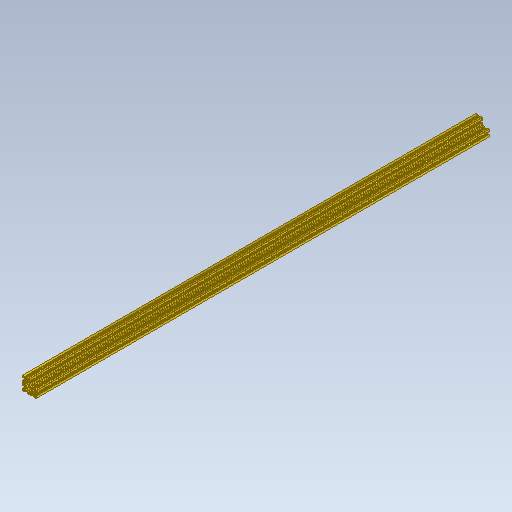
# Autodesk Inventor part: Perfil 60×60 L 8 rasgos_AST060060L08
Saved by Autodesk Inventor 2025.2 (Build 292293000, 293)
## iProperties
Created: 2025-04-07
Part Number: Perfil 60×60 L 8 rasgos_AST060060L08
Material: Ouro
Document SubType Name: Modeling
Designer: Gustavo Sousa
Density: 19.3 g/cm^3
Appearance: Metal quente 2400F
Author: Gustavo Sousa
Autodesk Inventor part; units mm, degrees
ref_plane "YZ Plane" through (0, 0, 0) normal (1, 0, 0) x (0, 1, 0)
ref_plane "XZ Plane" through (0, 0, 0) normal (0, 1, 0) x (-1, 0, 0)
ref_plane "XY Plane" through (0, 0, 0) normal (0, 0, 1) x (1, 0, 0)
sketch "Esboço1" plane through (0, 0, 0) normal (0, 0, 1) x (1, 0, 0)
  line L0 (-30, 30) -> (30, 30) construction
  line L1 (-30, 30) -> (-30, -30) construction
  line L2 (-30, -30) -> (30, -30) construction
  line L3 (30, 30) -> (30, -30) construction
  circle A0 centre (-15, 15) radius 5
  line L4 (-15, 15) -> (0, 0) construction
  line L5 (-15, 15) -> (0, 30) construction
  line L6 (-15, 15) -> (-30, 30) construction
  line L7 (-15, 15) -> (-30, 0) construction
  circle A1 centre (-26.5, 26.5) radius 2.25
  arc A2 (-29.5, 30) -> (-30, 29.5) centre (-29.5, 29.5) ccw
  line L8 (-22, 22) -> (-8, 22) construction
  line L9 (-19.1, 30) -> (-10.9, 30) construction
  line L10 (-19.1, 30) -> (-19.6, 30) construction
  line L11 (-19.6, 30) -> (-19.6, 29.5)
  line L12 (-19.6, 29.5) -> (-19.1, 29.5)
  line L13 (-19.1, 29.5) -> (-19.1, 30) construction
  line L14 (-19.6, 30) -> (-29.5, 30)
  line L15 (-19.1, 30) -> (-19.1, 27.8) construction
  line L16 (-19.1, 27.8) -> (-23.15, 27.8)
  line L17 (-19.1, 29.5) -> (-19.1, 27.8)
  line L18 (-22, 22) -> (-22, 8) construction
  line L19 (-23.15, 27.8) -> (-23.15, 24.7056)
  line L20 (-23.15, 24.7056) -> (-20.4444, 22)
  line L21 (-20.4444, 22) -> (-15, 22)
  line L22 (-8, 22) -> (-8, 8) construction
  line L23 (-22, 8) -> (-8, 8) construction
  line L24 (-30, 19.1) -> (-30, 10.9) construction
  line L25 (-10.9, 30) -> (-10.4, 30) construction
  line L26 (-10.4, 30) -> (-10.4, 29.5)
  line L27 (-10.4, 29.5) -> (-10.9, 29.5)
  line L28 (-10.9, 29.5) -> (-10.9, 30) construction
  arc A3 (0, 29.5) -> (-0.5, 30) centre (-0.5, 29.5) ccw
  line L29 (0, 30) -> (0, 0) construction
  line L30 (-10.4, 30) -> (-0.5, 30)
  line L31 (-10.9, 30) -> (-10.9, 27.8) construction
  line L32 (-10.9, 27.8) -> (-6.85, 27.8)
  line L33 (-6.85, 27.8) -> (-6.85, 24.7056)
  line L34 (-6.85, 24.7056) -> (-9.5556, 22)
  line L35 (-9.5556, 22) -> (-15, 22)
  circle A4 centre (-3.5, 26.5) radius 2.25
  line L36 (-30, 19.1) -> (-29.5, 19.1) construction
  line L37 (-29.5, 19.1) -> (-29.5, 19.6)
  line L38 (-29.5, 19.6) -> (-30, 19.6)
  line L39 (-30, 19.6) -> (-30, 19.1) construction
  line L40 (-30, 10.9) -> (-29.5, 10.9) construction
  line L41 (-29.5, 10.9) -> (-29.5, 10.4)
  line L42 (-29.5, 10.4) -> (-30, 10.4)
  line L43 (-30, 10.4) -> (-30, 10.9) construction
  line L44 (-10.9, 29.5) -> (-10.9, 27.8)
  line L45 (-30, 19.6) -> (-30, 29.5)
  line L46 (-30, 19.1) -> (-27.8, 19.1) construction
  line L47 (-27.8, 23.15) -> (-27.8, 19.1)
  line L48 (-27.8, 23.15) -> (-24.7056, 23.15)
  line L49 (-24.7056, 23.15) -> (-22, 20.4444)
  line L50 (-29.5, 19.1) -> (-27.8, 19.1)
  line L51 (-22, 20.4444) -> (-22, 15)
  line L52 (-30, 10.4) -> (-30, 0)
  line L53 (-30, 10.9) -> (-27.8, 10.9) construction
  line L54 (-27.8, 10.9) -> (-27.8, 6.85)
  line L55 (-27.8, 6.85) -> (-24.7056, 6.85)
  line L56 (-24.7056, 6.85) -> (-22, 9.5556)
  line L57 (-22, 15) -> (-22, 9.5556)
  line L58 (-29.5, 10.9) -> (-27.8, 10.9)
  line L59 (-30, 0) -> (-27.8, 0) construction
  line L60 (-27.8, 0) -> (-27.8, 4.65)
  line L61 (-20.4444, 8) -> (-23.7944, 4.65)
  line L62 (-27.8, 4.65) -> (-23.7944, 4.65)
  line L63 (0, 19.1) -> (0, 10.9) construction
  line L64 (0, 19.1) -> (-0.5, 19.1) construction
  line L65 (-0.5, 19.1) -> (-0.5, 19.6)
  line L66 (-0.5, 19.6) -> (0, 19.6)
  line L67 (0, 19.6) -> (0, 19.1) construction
  line L68 (0, 10.9) -> (-0.5, 10.9) construction
  line L69 (-0.5, 10.9) -> (-0.5, 10.4)
  line L70 (-0.5, 10.4) -> (0, 10.4)
  line L71 (0, 10.4) -> (0, 10.9) construction
  line L72 (0, 19.6) -> (0, 29.5)
  line L73 (-2.2, 19.1) -> (0, 19.1) construction
  line L74 (-2.2, 19.1) -> (-2.2, 23.15)
  line L75 (-5.2944, 23.15) -> (-2.2, 23.15)
  line L76 (-5.2944, 23.15) -> (-8, 20.4444)
  line L77 (-2.2, 19.1) -> (-0.5, 19.1)
  line L78 (-8, 20.4444) -> (-8, 15)
  line L79 (-2.2, 10.9) -> (0, 10.9) construction
  line L80 (-2.2, 10.9) -> (-2.2, 6.85)
  line L81 (-2.2, 6.85) -> (-5.2944, 6.85)
  line L82 (-8, 9.5556) -> (-5.2944, 6.85)
  line L83 (-8, 9.5556) -> (-8, 15)
  line L84 (-2.2, 10.9) -> (-0.5, 10.9)
  line L85 (-20.4444, 8) -> (-15, 8)
  line L86 (0, 10.4) -> (0, 0)
  line L87 (0, 0) -> (-2.2, 0) construction
  line L88 (-2.2, 4.65) -> (-2.2, 0)
  line L89 (-6.2056, 4.65) -> (-2.2, 4.65)
  line L90 (-9.5556, 8) -> (-6.2056, 4.65)
  line L91 (-15, 8) -> (-9.5556, 8)
  circle A5 centre (-18.5355, 18.5355) radius 1.1
  circle A6 centre (-18.5355, 11.4645) radius 1.1
  circle A7 centre (-11.4645, 11.4645) radius 1.1
  circle A8 centre (-11.4645, 18.5355) radius 1.1
  circle A9 centre (-15, -15) radius 5
  line L92 (-15, -15) -> (-30, 0) construction
  line L93 (-15, -15) -> (-30, -30) construction
  line L94 (-15, -15) -> (0, 0) construction
  line L95 (-15, -15) -> (0, -30) construction
  line L96 (-30, 0) -> (-30, -30) construction
  line L97 (0, 0) -> (0, -30) construction
  line L98 (-22, -8) -> (-22, -22) construction
  line L99 (-22, -8) -> (-8, -8) construction
  line L100 (-8, -8) -> (-8, -22) construction
  line L101 (-8, -22) -> (-22, -22) construction
  line L102 (-30, -10.9) -> (-30, -19.1) construction
  line L103 (-27.8, 0) -> (-27.8, -4.65)
  line L104 (-27.8, -4.65) -> (-23.7944, -4.65)
  line L105 (-23.7944, -4.65) -> (-20.4444, -8)
  line L106 (-30, -10.9) -> (-29.5, -10.9) construction
  line L107 (-29.5, -10.9) -> (-29.5, -10.4)
  line L108 (-29.5, -10.4) -> (-30, -10.4)
  line L109 (-30, -10.4) -> (-30, -10.9) construction
  line L110 (-30, -19.1) -> (-29.5, -19.1) construction
  line L111 (-29.5, -19.1) -> (-29.5, -19.6)
  line L112 (-29.5, -19.6) -> (-30, -19.6)
  line L113 (-30, -19.6) -> (-30, -19.1) construction
  line L114 (-30, 0) -> (-30, -10.4)
  line L115 (-30, -10.9) -> (-27.8, -10.9) construction
  line L116 (-27.8, -10.9) -> (-27.8, -6.85)
  line L117 (-27.8, -6.85) -> (-24.7056, -6.85)
  line L118 (-24.7056, -6.85) -> (-22, -9.5556)
  line L119 (-22, -9.5556) -> (-22, -15)
  arc A10 (-30, -29.5) -> (-29.5, -30) centre (-29.5, -29.5) ccw
  line L120 (-30, -19.6) -> (-30, -29.5)
  line L121 (-30, -19.1) -> (-27.8, -19.1) construction
  line L122 (-27.8, -19.1) -> (-27.8, -23.15)
  line L123 (-27.8, -23.15) -> (-24.7056, -23.15)
  line L124 (-24.7056, -23.15) -> (-22, -20.4444)
  line L125 (-22, -15) -> (-22, -20.4444)
  line L126 (-29.5, -19.1) -> (-27.8, -19.1)
  circle A11 centre (-26.5, -26.5) radius 2.25
  line L127 (-2.2, 0) -> (-10.2, -8)
  line L128 (-20.4444, -8) -> (-15, -8)
  line L129 (-10.2, -8) -> (-15, -8)
  line L130 (-29.5, -10.9) -> (-27.8, -10.9)
  line L131 (-19.1, -30) -> (-10.9, -30) construction
  line L132 (-19.1, -30) -> (-19.6, -30) construction
  line L133 (-19.6, -30) -> (-19.6, -29.5)
  line L134 (-19.6, -29.5) -> (-19.1, -29.5)
  line L135 (-19.1, -29.5) -> (-19.1, -30) construction
  line L136 (-10.9, -30) -> (-10.4, -30) construction
  line L137 (-10.4, -30) -> (-10.4, -29.5)
  line L138 (-10.4, -29.5) -> (-10.9, -29.5)
  line L139 (-10.9, -29.5) -> (-10.9, -30) construction
  line L140 (-19.6, -30) -> (-29.5, -30)
  line L141 (-19.1, -27.8) -> (-19.1, -30) construction
  line L142 (-19.1, -27.8) -> (-23.15, -27.8)
  line L143 (-23.15, -24.7056) -> (-23.15, -27.8)
  line L144 (-23.15, -24.7056) -> (-20.4444, -22)
  line L145 (-19.1, -27.8) -> (-19.1, -29.5)
  line L146 (-20.4444, -22) -> (-15, -22)
  line L147 (-10.4, -30) -> (0, -30)
  line L148 (-10.9, -27.8) -> (-10.9, -30) construction
  line L149 (-10.9, -27.8) -> (-6.85, -27.8)
  line L150 (-10.9, -27.8) -> (-10.9, -29.5)
  line L151 (-6.85, -24.7056) -> (-6.85, -27.8)
  line L152 (-9.5556, -22) -> (-6.85, -24.7056)
  line L153 (-15, -22) -> (-9.5556, -22)
  circle A12 centre (-18.5355, -11.4645) radius 1.1
  circle A13 centre (-18.5355, -18.5355) radius 1.1
  circle A14 centre (-11.4645, -18.5355) radius 1.1
  circle A15 centre (-11.4645, -11.4645) radius 1.1
  line L154 (-8, -9.5556) -> (-0.6444, -2.2)
  line L155 (0, 0) -> (30, 0) construction
  line L156 (-8, -20.4444) -> (-4.65, -23.7944)
  line L157 (-8, -9.5556) -> (-8, -20.4444)
  line L158 (-4.65, -23.7944) -> (-4.65, -27.8)
  line L159 (0, -30) -> (0, -27.8) construction
  line L160 (0, -27.8) -> (-4.65, -27.8)
  line L161 (-0.6444, -2.2) -> (0, -2.2)
  line L162 (0, -30) -> (30, -30) construction
  circle A16 centre (15, -15) radius 5
  line L163 (15, -15) -> (0, -30) construction
  line L164 (15, -15) -> (0, 0) construction
  line L165 (15, -15) -> (30, 0) construction
  line L166 (15, -15) -> (30, -30) construction
  line L167 (10.9, -30) -> (19.1, -30) construction
  line L168 (10.9, -30) -> (10.4, -30) construction
  line L169 (10.4, -30) -> (10.4, -29.5)
  line L170 (10.4, -29.5) -> (10.9, -29.5)
  line L171 (10.9, -29.5) -> (10.9, -30) construction
  line L172 (19.1, -30) -> (19.6, -30) construction
  line L173 (19.6, -30) -> (19.6, -29.5)
  line L174 (19.6, -29.5) -> (19.1, -29.5)
  line L175 (19.1, -29.5) -> (19.1, -30) construction
  line L176 (0, -30) -> (10.4, -30)
  line L177 (10.9, -27.8) -> (10.9, -30) construction
  line L178 (10.9, -27.8) -> (6.85, -27.8)
  line L179 (10.9, -27.8) -> (10.9, -29.5)
  line L180 (6.85, -24.7056) -> (6.85, -27.8)
  line L181 (8, -22) -> (22, -22) construction
  line L182 (6.85, -24.7056) -> (9.5556, -22)
  line L183 (9.5556, -22) -> (15, -22)
  line L184 (19.1, -27.8) -> (19.1, -30) construction
  line L185 (19.1, -27.8) -> (23.15, -27.8)
  line L186 (23.15, -24.7056) -> (23.15, -27.8)
  line L187 (20.4444, -22) -> (23.15, -24.7056)
  line L188 (20.4444, -22) -> (15, -22)
  circle A17 centre (26.5, -26.5) radius 2.25
  line L189 (19.1, -29.5) -> (19.1, -27.8)
  line L190 (8, -22) -> (8, -8) construction
  line L191 (8, -8) -> (22, -8) construction
  line L192 (22, -8) -> (22, -22) construction
  line L193 (0, -27.8) -> (4.65, -27.8)
  line L194 (4.65, -23.7944) -> (4.65, -27.8)
  line L195 (4.65, -23.7944) -> (8, -20.4444)
  arc A18 (29.5, -30) -> (30, -29.5) centre (29.5, -29.5) ccw
  line L196 (19.6, -30) -> (29.5, -30)
  line L197 (8, -20.4444) -> (8, -15)
  line L198 (30, -10.9) -> (30, -19.1) construction
  line L199 (30, -19.1) -> (29.5, -19.1) construction
  line L200 (29.5, -19.1) -> (29.5, -19.6)
  line L201 (29.5, -19.6) -> (30, -19.6)
  line L202 (30, -19.6) -> (30, -19.1) construction
  line L203 (30, -10.9) -> (29.5, -10.9) construction
  line L204 (29.5, -10.9) -> (29.5, -10.4)
  line L205 (29.5, -10.4) -> (30, -10.4)
  line L206 (30, -10.4) -> (30, -10.9) construction
  line L207 (30, -19.6) -> (30, -29.5)
  line L208 (27.8, -19.1) -> (30, -19.1) construction
  line L209 (27.8, -19.1) -> (27.8, -23.15)
  line L210 (27.8, -23.15) -> (24.7056, -23.15)
  line L211 (22, -20.4444) -> (24.7056, -23.15)
  line L212 (27.8, -19.1) -> (29.5, -19.1)
  line L213 (22, -20.4444) -> (22, -15)
  arc A19 (30, -0.5) -> (29.5, 0) centre (29.5, -0.5) ccw
  line L214 (30, -0.5) -> (30, -10.4)
  line L215 (27.8, -10.9) -> (30, -10.9) construction
  line L216 (27.8, -6.85) -> (27.8, -10.9)
  line L217 (24.7056, -6.85) -> (27.8, -6.85)
  line L218 (24.7056, -6.85) -> (22, -9.5556)
  line L219 (22, -9.5556) -> (22, -15)
  line L220 (27.8, -10.9) -> (29.5, -10.9)
  line L221 (10.9, 0) -> (19.1, 0)
  line L222 (19.1, 0) -> (19.6, 0) construction
  line L223 (19.6, 0) -> (19.6, -0.5)
  line L224 (19.6, -0.5) -> (19.1, -0.5)
  line L225 (19.1, -0.5) -> (19.1, 0) construction
  line L226 (10.9, 0) -> (10.4, 0) construction
  line L227 (10.4, 0) -> (10.4, -0.5)
  line L228 (10.4, -0.5) -> (10.9, -0.5)
  line L229 (10.9, -0.5) -> (10.9, 0) construction
  line L230 (0, 0) -> (10.4, 0)
  line L231 (10.9, 0) -> (10.9, -2.2) construction
  line L232 (10.9, -2.2) -> (6.85, -2.2)
  line L233 (6.85, -2.2) -> (6.85, -5.2944)
  line L234 (6.85, -5.2944) -> (9.5556, -8)
  line L235 (9.5556, -8) -> (15, -8)
  line L236 (19.1, 0) -> (19.1, -2.2) construction
  line L237 (19.1, -2.2) -> (23.15, -2.2)
  line L238 (23.15, -2.2) -> (23.15, -5.2944)
  line L239 (23.15, -5.2944) -> (20.4444, -8)
  line L240 (20.4444, -8) -> (15, -8)
  line L241 (10.9, -0.5) -> (10.9, -2.2)
  line L242 (19.1, -0.5) -> (19.1, -2.2)
  line L243 (19.6, 0) -> (29.5, 0)
  circle A20 centre (26.5, -3.5) radius 2.25
  line L244 (0, -2.2) -> (4.65, -2.2)
  line L245 (4.65, -2.2) -> (4.65, -6.2056)
  line L246 (4.65, -6.2056) -> (8, -9.5556)
  line L247 (8, -9.5556) -> (8, -15)
  circle A21 centre (11.4645, -11.4645) radius 1.1
  circle A22 centre (11.4645, -18.5355) radius 1.1
  circle A23 centre (18.5355, -18.5355) radius 1.1
  circle A24 centre (18.5355, -11.4645) radius 1.1
  point P0 (-15, 30)
  point P1 (-30, 15)
  point P2 (0, 15)
  point P3 (0, 15)
  point P4 (0, -15)
  point P5 (-30, -15)
  point P6 (-30, -15)
  point P7 (-15, -30)
  point P8 (-12.3231, 19.2231)
  point P9 (-10.7769, 17.6769)
  point P10 (-10.7769, 12.3231)
  point P11 (-12.3231, 10.7769)
  point P12 (-17.6769, 10.7769)
  point P13 (-19.2231, 12.3231)
  point P14 (-19.2231, 17.6769)
  point P15 (-17.6769, 19.2231)
  point P16 (-12.3231, -10.7769)
  point P17 (-10.7769, -12.3231)
  point P18 (-10.7769, -17.6769)
  point P19 (-12.3231, -19.2231)
  point P20 (-17.6769, -19.2231)
  point P21 (-19.2231, -17.6769)
  point P22 (-19.2231, -12.3231)
  point P23 (-17.6769, -10.7769)
  point P24 (15, 0)
  point P25 (15, -30)
  point P26 (15, -30)
  point P27 (30, -15)
  point P28 (15, 0)
  point P29 (17.6769, -10.7769)
  point P30 (19.2231, -12.3231)
  point P31 (19.2231, -17.6769)
  point P32 (17.6769, -19.2231)
  point P33 (12.3231, -19.2231)
  point P34 (10.7769, -17.6769)
  point P35 (10.7769, -12.3231)
  point P36 (12.3231, -10.7769)
  dimension "d4" = 10
  dimension "d0" = 60
  dimension "d3" = 15
  dimension "d5" = 26.5
  dimension "d7" = 4.5
  dimension "arco" = 0.5
  dimension "d9" = 8
  dimension "d10" = 8.2
  dimension "quadrado" = 0.5
  dimension "espessura" = 2.2
  dimension "d14" = 1.1
  dimension "d16" = 1.1
  dimension "d18" = 1.1
  dimension "d20" = 2.2
  dimension "d21" = 2.2
  dimension "d24" = 360
  dimension "d27" = 8
  dimension "d32" = 360
  dimension "d34" = 1.1
  dimension "d35" = 1.1
  dimension "d36" = 2.2
  dimension "d37" = 2.2
  dimension "d41" = 8
  dimension "d45" = 360
  constraints: 496 end point, 104 equal length, 56 parallel, 54 horizontal, 45 point on line, 39 collinear, 39 vertical, 28 midpoint, 25 perpendicular, 22 centre point, 13 vertical alignment, 12 horizontal alignment, 10 equal radius, 10 point on circle, 10 tangent, 6 coincident, 36 other
  measures "d0" distance of L0.start L0.end
  measures "d3" horizontal distance of L4.end L4.start
  measures "d5" horizontal distance of L4.end A1.centre
  measures "d7" diameter of A1
  measures "arco" radius of A2
  measures "d9" distance between parallel lines of L0 L8
  measures "d10" distance of L9.start L9.end
  measures "quadrado" distance of L12.end L9.start
  measures "espessura" distance between parallel lines of L16 L0
  measures "d14" distance edge to line of A1 L19
  measures "d16" distance between parallel lines of L6 L20
  measures "d18" distance between parallel lines of L7 L61
  measures "d20" distance between parallel lines of L62 L55
  measures "d21" diameter of A5
  measures "d27" distance between parallel lines of L1 L98
  measures "d34" distance between parallel lines of L94 L154
  measures "d35" distance between parallel lines of L95 L156
  measures "d36" distance between parallel lines of L151 L158
  measures "d37" distance between parallel lines of L155 L161
  measures "d41" distance from line of point (15, -30) L181
extrude "Extrusão2" add sketch "Esboço1" along normal mid plane 2000
fillet "Arredondamento1" radius 1 70 edges at (-24.7056, -6.85, 0) (-22, -9.5556, 0) (-27.8, -6.85, 0) (-22, -20.4444, 0) (-24.7056, -23.15, 0) (-27.8, -23.15, 0) (-23.15, -27.8, 0) (-23.15, -24.7056, 0) (-20.4444, -22, 0) (-9.5556, -22, 0) (-6.85, -24.7056, 0) (-6.85, -27.8, 0) (-27.8, -4.65, 0) (-23.7944, -4.65, 0) (-20.4444, -8, 0) (-27.8, 4.65, 0) (-23.7944, 4.65, 0) (-20.4444, 8, 0) (-10.2, -8, 0) (-9.5556, 8, 0) (-6.2056, 4.65, 0) (-2.2, 4.65, 0) (-2.2, 0, 0) (-27.8, 23.15, 0) (-24.7056, 23.15, 0) (-22, 20.4444, 0) (-24.7056, 6.85, 0) (-22, 9.5556, 0) (-27.8, 6.85, 0) (-6.85, 24.7056, 0) (-9.5556, 22, 0) (-6.85, 27.8, 0) (-23.15, 24.7056, 0) (-20.4444, 22, 0) (-23.15, 27.8, 0) (-2.2, 23.15, 0) (-2.2, 6.85, 0) (-5.2944, 6.85, 0) (-8, 9.5556, 0) (-5.2944, 23.15, 0) (-8, 20.4444, 0) (-4.65, -23.7944, 0) (-4.65, -27.8, 0) (-8, -20.4444, 0) (-8, -9.5556, 0) (-0.6444, -2.2, 0) (4.65, -6.2056, 0) (4.65, -2.2, 0) (8, -9.5556, 0) (8, -20.4444, 0) (4.65, -23.7944, 0) (4.65, -27.8, 0) (6.85, -2.2, 0) (6.85, -5.2944, 0) (9.5556, -8, 0) (20.4444, -8, 0) (23.15, -5.2944, 0) (23.15, -2.2, 0) (9.5556, -22, 0) (6.85, -24.7056, 0) (6.85, -27.8, 0) (20.4444, -22, 0) (23.15, -24.7056, 0) (23.15, -27.8, 0) (27.8, -23.15, 0) (24.7056, -23.15, 0) (22, -20.4444, 0) (27.8, -6.85, 0) (22, -9.5556, 0) (24.7056, -6.85, 0)
